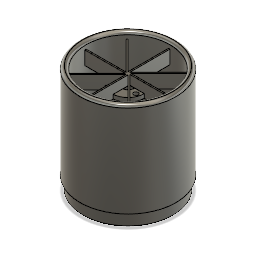
top v6 (Autodesk Fusion 360 design; units mm, degrees)
Autodesk Fusion 360 part; units mm, degrees
note: some values were not read from the file. Set by a fixed rule: which sketch regions a step uses.
sketch "草图1" plane through (0, 0, 0) normal (0, 1, 0) x (1, 0, 0)
  circle A0 centre (0, 0) radius 35.5
  dimension "d1" = 71
  measures "d1" diameter of A0
extrude "拉伸1" add sketch "草图1" along normal blind 80
sketch "草图2" plane through (0, 80, 0) normal (0, 1, 0) x (-1, 0, 0)
  circle A0 centre (0, 0) radius 35.5
  circle A1 centre (0, 0) radius 31
  dimension "d4" = 62
  measures "d4" diameter of A1
extrude "拉伸2" cut sketch "草图2" against normal blind 90 contours A1
ref_plane "WorkPlane2" through (0, 75, 0) normal (0, 1, 0) x (-1, 0, 0)
sketch "Sketch5" plane through (0, 75, 0) normal (0, 1, 0) x (1, 0, 0)
  line L0 (0, 0) -> (31, 0)
  line L1 (31, 0) -> (31, 1)
  line L2 (31, 1) -> (0, 1)
  line L3 (0, 1) -> (0, 0)
  circle A0 centre (0, 0) radius 35.5
  circle A1 centre (0, 0) radius 35.5
  circle A2 centre (0, 0) radius 31
  dimension "d18" = 1
  measures "d18" distance of L0 L2
extrude "Extrude5" add sketch "Sketch5" against normal blind 10 contours L0 L2 L3 A2 picked at (10.328, 0.6667)
pattern_circular "C-Pattern1" count 8 over 360 about axis through (0, 1.75, 0) along (0, 1, 0) of "Extrude5"
sketch "Sketch6" plane through (0, 65, 0) normal (0, -1, 0) x (1, 0, 0)
  line L0 (1.4142, 0) -> (22.616, 21.2018)
  arc A0 (22.616, 21.2018) -> (21.9203, 21.9203) centre (0, 0) ccw
  line L1 (21.9203, 21.9203) -> (1, 1)
  line L2 (1, 1) -> (1, 30.9839)
  arc A1 (1, 30.9839) -> (0, 31) centre (0, 0) ccw
  line L3 (0, 31) -> (0, 1.4142)
  line L4 (0, 1.4142) -> (-21.2018, 22.616)
  arc A2 (-21.2018, 22.616) -> (-21.9203, 21.9203) centre (0, 0) ccw
  line L5 (-21.9203, 21.9203) -> (-1, 1)
  line L6 (-1, 1) -> (-30.9839, 1)
  arc A3 (-30.9839, 1) -> (-31, 0) centre (0, 0) ccw
  line L7 (-31, 0) -> (-1.4142, 0)
  line L8 (-1.4142, 0) -> (-22.616, -21.2018)
  arc A4 (-22.616, -21.2018) -> (-21.9203, -21.9203) centre (0, 0) ccw
  line L9 (-21.9203, -21.9203) -> (-1, -1)
  line L10 (-1, -1) -> (-1, -30.9839)
  arc A5 (-1, -30.9839) -> (0, -31) centre (0, 0) ccw
  line L11 (0, -31) -> (0, -1.4142)
  line L12 (0, -1.4142) -> (21.2018, -22.616)
  arc A6 (21.2018, -22.616) -> (21.9203, -21.9203) centre (0, 0) ccw
  line L13 (21.9203, -21.9203) -> (1, -1)
  line L14 (1, -1) -> (30.9839, -1)
  arc A7 (30.9839, -1) -> (31, 0) centre (0, 0) ccw
  line L15 (31, 0) -> (1.4142, 0)
  circle A8 centre (0, 0) radius 12
  dimension "d23" = 24
  measures "d23" diameter of A8
extrude "Extrude6" add sketch "Sketch6" against normal blind 3 contours L0 L1 L2 L3 L4 L5 L6 L7 L8 L9 L10 L11 L12 L13 L14 L15 A8 | L0 L15 A8 | L1 L2 A8 | L13 L14 A8 | L3 L4 A8 | L11 L12 A8 | L5 L6 A8 | L9 L10 A8 | L7 L8 A8
sketch "Sketch7" plane through (0, 65, 0) normal (0, -1, 0) x (1, 0, 0)
  line L0 (9.1629, 7.7487) -> (22.616, 21.2018)
  arc A0 (22.616, 21.2018) -> (21.9203, 21.9203) centre (0, 0) ccw
  line L1 (21.9203, 21.9203) -> (8.4853, 8.4853)
  arc A1 (8.4853, 8.4853) -> (1, 11.9583) centre (0, 0) ccw
  line L2 (1, 11.9583) -> (1, 30.9839)
  arc A2 (1, 30.9839) -> (0, 31) centre (0, 0) ccw
  line L3 (0, 31) -> (0, 12)
  arc A3 (0, 12) -> (-7.7487, 9.1629) centre (0, 0) ccw
  line L4 (-7.7487, 9.1629) -> (-21.2018, 22.616)
  arc A4 (-21.2018, 22.616) -> (-21.9203, 21.9203) centre (0, 0) ccw
  line L5 (-21.9203, 21.9203) -> (-8.4853, 8.4853)
  arc A5 (-8.4853, 8.4853) -> (-11.9583, 1) centre (0, 0) ccw
  line L6 (-11.9583, 1) -> (-30.9839, 1)
  arc A6 (-30.9839, 1) -> (-31, 0) centre (0, 0) ccw
  line L7 (-31, 0) -> (-12, 0)
  arc A7 (-12, 0) -> (-9.1629, -7.7487) centre (0, 0) ccw
  line L8 (-9.1629, -7.7487) -> (-22.616, -21.2018)
  arc A8 (-22.616, -21.2018) -> (-21.9203, -21.9203) centre (0, 0) ccw
  line L9 (-21.9203, -21.9203) -> (-8.4853, -8.4853)
  arc A9 (-8.4853, -8.4853) -> (-1, -11.9583) centre (0, 0) ccw
  line L10 (-1, -11.9583) -> (-1, -30.9839)
  arc A10 (-1, -30.9839) -> (0, -31) centre (0, 0) ccw
  arc A11 (0, -12) -> (7.7487, -9.1629) centre (0, 0) ccw
  line L11 (7.7487, -9.1629) -> (21.2018, -22.616)
  arc A12 (21.2018, -22.616) -> (21.9203, -21.9203) centre (0, 0) ccw
  line L12 (21.9203, -21.9203) -> (8.4853, -8.4853)
  arc A13 (8.4853, -8.4853) -> (11.9583, -1) centre (0, 0) ccw
  line L13 (11.9583, -1) -> (30.9839, -1)
  arc A14 (30.9839, -1) -> (31, 0) centre (0, 0) ccw
  arc A15 (12, 0) -> (9.1629, 7.7487) centre (0, 0) ccw
  circle A16 centre (0, 0) radius 5
  line L14 (0, -31) -> (0, -12)
  line L15 (31, 0) -> (12, 0)
  dimension "d26" = 10
  measures "d26" diameter of A16
extrude "Extrude7" cut sketch "Sketch7" against normal blind 3 contours A16
sketch "Sketch8" plane through (0, 65, 0) normal (0, -1, 0) x (1, 0, 0)
  circle A0 centre (0, 0) radius 5
  line L0 (9.1629, 7.7487) -> (22.616, 21.2018)
  arc A1 (22.616, 21.2018) -> (21.9203, 21.9203) centre (0, 0) ccw
  line L1 (21.9203, 21.9203) -> (8.4853, 8.4853)
  arc A2 (8.4853, 8.4853) -> (1, 11.9583) centre (0, 0) ccw
  line L2 (1, 11.9583) -> (1, 30.9839)
  arc A3 (1, 30.9839) -> (0, 31) centre (0, 0) ccw
  line L3 (0, 31) -> (0, 12)
  arc A4 (0, 12) -> (-7.7487, 9.1629) centre (0, 0) ccw
  line L4 (-7.7487, 9.1629) -> (-21.2018, 22.616)
  arc A5 (-21.2018, 22.616) -> (-21.9203, 21.9203) centre (0, 0) ccw
  line L5 (-21.9203, 21.9203) -> (-8.4853, 8.4853)
  arc A6 (-8.4853, 8.4853) -> (-11.9583, 1) centre (0, 0) ccw
  line L6 (-11.9583, 1) -> (-30.9839, 1)
  arc A7 (-30.9839, 1) -> (-31, 0) centre (0, 0) ccw
  line L7 (-31, 0) -> (-12, 0)
  arc A8 (-12, 0) -> (-9.1629, -7.7487) centre (0, 0) ccw
  line L8 (-9.1629, -7.7487) -> (-22.616, -21.2018)
  arc A9 (-22.616, -21.2018) -> (-21.9203, -21.9203) centre (0, 0) ccw
  line L9 (-21.9203, -21.9203) -> (-8.4853, -8.4853)
  arc A10 (-8.4853, -8.4853) -> (-1, -11.9583) centre (0, 0) ccw
  line L10 (-1, -11.9583) -> (-1, -30.9839)
  arc A11 (-1, -30.9839) -> (0, -31) centre (0, 0) ccw
  arc A12 (0, -12) -> (7.7487, -9.1629) centre (0, 0) ccw
  line L11 (7.7487, -9.1629) -> (21.2018, -22.616)
  arc A13 (21.2018, -22.616) -> (21.9203, -21.9203) centre (0, 0) ccw
  line L12 (21.9203, -21.9203) -> (8.4853, -8.4853)
  arc A14 (8.4853, -8.4853) -> (11.9583, -1) centre (0, 0) ccw
  line L13 (11.9583, -1) -> (30.9839, -1)
  arc A15 (30.9839, -1) -> (31, 0) centre (0, 0) ccw
  arc A16 (12, 0) -> (9.1629, 7.7487) centre (0, 0) ccw
  line L14 (-42.8424, -14.7518) -> (51.2572, 17.6493) construction
  line L15 (-13.299, 38.6232) -> (13.2323, -38.4293) construction
  circle A17 centre (0, 0) radius 9.5 construction
  circle A18 centre (0, 0) radius 8 construction
  line L16 (0, -31) -> (0, -12)
  line L17 (31, 0) -> (12, 0)
  dimension "d29" = 90
  dimension "d31" = 19
  dimension "d32" = 16
  measures "d29" angle of L14 L15
  measures "d31" diameter of A17
  measures "d32" diameter of A18
hole "Hole1" at (-2.6045, 65, 7.5641) at (8.9824, 65, 3.0929) at (2.6045, 65, -7.5641) at (-8.9824, 65, -3.0929) direction (0, 1, 0) diameter 3.4 depth 3 tip angle 118
fillet "Fillet2" radius 2.2 2 edges at (-33.0976, 80, 12.8373) (28.9021, 80, 11.2101)
sketch "Sketch9" plane through (0, 0, 0) normal (0, -1, 0) x (1, 0, 0)
  circle A0 centre (0, 0) radius 31
  circle A1 centre (0, 0) radius 35.5
  circle A2 centre (0, 0) radius 33.5
  dimension "d45" = 67
  measures "d45" diameter of A2
extrude "Extrude8" cut sketch "Sketch9" against normal blind 10 contours A1
chamfer "Chamfer1" distance 1 angle 45 1 edges at (-31.233, 0, -12.1141)
